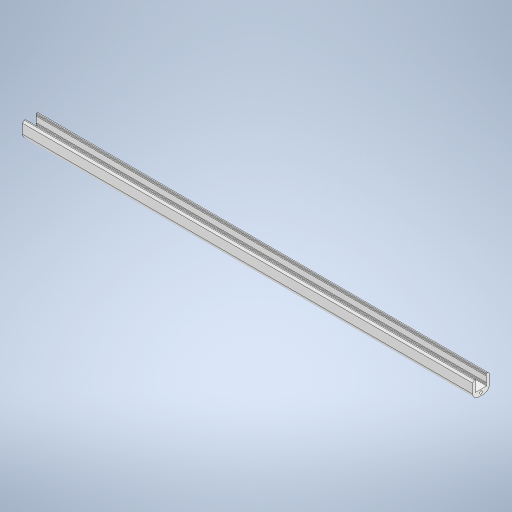
# Autodesk Inventor part: Nomad Slot Filler
Saved by Autodesk Inventor 2023.2 (Build 272271000, 271)
## iProperties
Created: 2023-06-29
Part Number: Nomad Slot Filler
Material: Silicon Nitride
Document SubType Name: Modeling
Designer: Nathan Cai
Density: 3.18 g/cm^3
Appearance: Smooth - White
Author: Nathan Cai
Autodesk Inventor part; units mm, degrees
ref_plane "YZ Plane" through (0, 0, 0) normal (1, 0, 0) x (0, 1, 0)
ref_plane "XZ Plane" through (0, 0, 0) normal (0, 1, 0) x (-1, 0, 0)
ref_plane "XY Plane" through (0, 0, 0) normal (0, 0, 1) x (1, 0, 0)
sketch "Sketch1" plane through (0, 0, 0) normal (1, 0, 0) x (0, 1, 0)
  line L0 (-1.5875, 1.5875) -> (1.5875, 1.5875)
  line L1 (1.5875, 1.5875) -> (1.5875, -1.5875) construction
  line L2 (1.5875, -1.5875) -> (-1.5875, -1.5875)
  line L3 (-1.5875, -1.5875) -> (-1.5875, 1.5875)
  line L4 (-1.5875, 1.5875) -> (1.5875, -1.5875) construction
  line L5 (1.5875, 1.5875) -> (-1.5875, -1.5875) construction
  line L6 (-1.5875, 2.3813) -> (1.5875, 2.3813)
  line L7 (1.5875, 2.3813) -> (1.5875, -2.3813)
  line L8 (1.5875, -2.3813) -> (-1.5875, -2.3813)
  line L9 (-1.5875, -2.3813) -> (-1.5875, 2.3813)
  line L10 (-1.5875, 2.3813) -> (1.5875, -2.3813) construction
  line L11 (1.5875, 2.3813) -> (-1.5875, -2.3813) construction
  line L12 (-1.5875, 2.3813) -> (-3.175, 2.3812)
  line L13 (-3.175, 2.3812) -> (-3.175, -2.3813)
  line L14 (-3.175, -2.3813) -> (-1.5875, -2.3813)
  line L15 (-1.5875, -2.3813) -> (-1.5875, 2.3813)
  line L16 (0.8083, 1.5875) -> (1.0583, 1.8375) construction
  line L17 (1.0583, 1.8375) -> (1.3083, 1.5875) construction
  line L18 (1.3083, 1.5875) -> (1.1998, 1.4789)
  line L19 (0.9169, 1.4789) -> (0.8083, 1.5875)
  line L20 (-0.8083, 1.5875) -> (-0.9169, 1.4789)
  line L21 (-1.1998, 1.4789) -> (-1.3083, 1.5875)
  line L22 (-1.3083, 1.5875) -> (-1.0583, 1.8375) construction
  line L23 (-1.0583, 1.8375) -> (-0.8083, 1.5875) construction
  line L24 (1.5875, 0) -> (-1.5875, 0) construction
  arc A0 (0.9169, 1.4789) -> (1.1998, 1.4789) centre (1.0583, 1.6203) ccw
  arc A1 (-1.1998, 1.4789) -> (-0.9169, 1.4789) centre (-1.0583, 1.6203) ccw
  line L25 (0.8083, -1.5875) -> (1.0583, -1.8375) construction
  line L26 (1.0583, -1.8375) -> (1.3083, -1.5875) construction
  line L27 (1.3083, -1.5875) -> (1.1998, -1.4789)
  line L28 (0.9169, -1.4789) -> (0.8083, -1.5875)
  line L29 (-0.8083, -1.5875) -> (-0.9169, -1.4789)
  line L30 (-1.1998, -1.4789) -> (-1.3083, -1.5875)
  line L31 (-1.3083, -1.5875) -> (-1.0583, -1.8375) construction
  line L32 (-1.0583, -1.8375) -> (-0.8083, -1.5875) construction
  arc A2 (1.1998, -1.4789) -> (0.9169, -1.4789) centre (1.0583, -1.6203) ccw
  arc A3 (-0.9169, -1.4789) -> (-1.1998, -1.4789) centre (-1.0583, -1.6203) ccw
  circle A4 centre (-2.3813, 0) radius 0.3969
  point P0 (0, 0)
  point P1 (1.0583, 1.5875)
  point P2 (1.0583, 1.3375)
  point P3 (-1.0583, 1.5875)
  point P4 (-1.0583, 1.3375)
  point P5 (1.0583, -1.5875)
  point P6 (1.0583, -1.3375)
  point P7 (-1.0583, -1.5875)
  point P8 (-1.0583, -1.3375)
  dimension "d0" = 3.175
  dimension "d1" = 3.175
  dimension "d2" = 3.175
  dimension "d3" = 4.7625
  dimension "d4" = 1.5875
  dimension "d5" = 0.5
  dimension "d6" = 0.5
  dimension "d7" = 0.2
  dimension "d14" = 0.7937
  dimension "d15" = 0.7937
  constraints: 66 end point, 16 point on line, 16 symmetric about line, 8 point on circle, 6 midpoint, 6 parallel, 5 centre point, 4 tangent, 3 horizontal, 3 perpendicular, 1 equal radius, 20 other
  measures "d0" distance of L1.end L2.end
  measures "d1" distance of L0.end L1.end
  measures "d2" distance of L7.end L8.end
  measures "d3" distance of L6.end L7.end
  measures "d4" distance of L14.end L13.end
  measures "d5" distance of L16.start L17.end
  measures "d6" distance of L21.end L20.start
  measures "d7" radius of A0
  measures "d14" diameter of A4
  measures "d15" distance from line of L3 A4.centre
extrude "Extrusion1" add sketch "Sketch1" along normal blind 127 contours L9 L6 L7 L0 | L3 L9 L14 L13 L12 | L0 L20 A1 L21 | L2 L7 L8 L9 | L30 A3 L29 L2 | L0 L18 A0 L19 | L28 A2 L27 L2
chamfer "Chamfer1" distance 0.5 angle 45 2 edges at (63.5, 1.5875, 2.3813) (63.5, 1.5875, -2.3813)
fillet "Fillet1" radius 1.5875 2 edges at (63.5, -3.175, 2.3812) (63.5, -3.175, -2.3813)
sketch "Sketch2" plane through (0, 1.0875, 2.3813) normal (0, 0, 1) x (1, 0, 0)
  line L0 (0, 0.1123) -> (127, 0.1123) projected
  line L1 (63.5, 0.1123) -> (63.5, -2.675)
  line L2 (0, -2.675) -> (127, -2.675) projected
  point P0 (0, -1.0875)
  constraints: 2 end point, 2 midpoint
equation "\"d6\" = d5"
equation "\"d15\" = 0.5 * d4"
body "Solid1"
